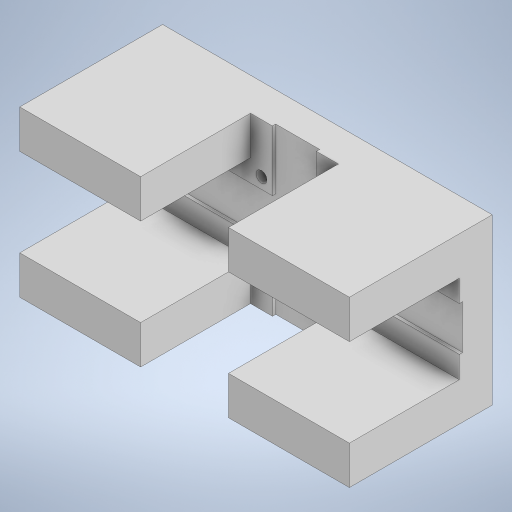
# Autodesk Inventor part: Bauteil1
Saved by Autodesk Inventor 2024 (Build 280153000, 153)
## iProperties
Created: 2023-11-13
Part Number: Bauteil1
Material: Generisch
Document SubType Name: Modeling
Designer: Luca
Density: 1 g/cm^3
Appearance: Vorgabe
Author: Luca
Autodesk Inventor part; units mm, degrees
ref_plane "YZ Plane" through (0, 0, 0) normal (1, 0, 0) x (0, 1, 0)
ref_plane "XZ Plane" through (0, 0, 0) normal (0, 1, 0) x (-1, 0, 0)
ref_plane "XY Plane" through (0, 0, 0) normal (0, 0, 1) x (1, 0, 0)
sketch "Skizze2" plane through (0, 0, 0) normal (0, 0, 1) x (1, 0, 0)
  line L0 (-30.3771, 139.6504) -> (269.6229, 139.6504)
  line L1 (269.6229, 139.6504) -> (269.6229, -10.3496)
  line L2 (269.6229, -10.3496) -> (-30.3771, -10.3496)
  line L3 (-30.3771, -10.3496) -> (-30.3771, 139.6504)
  point P0 (0, 0)
  dimension "d4" = 300
  dimension "d5" = 150
  constraints: 8 end point, 2 parallel, 1 horizontal, 1 perpendicular
  measures "d4" distance of L1.end L2.end
  measures "d5" distance between parallel lines of L2 L0
extrude "Extrusion2" add sketch "Skizze2" along normal blind 30
sketch "Skizze3" plane through (0, 0, 30) normal (0, 0, 1) x (1, 0, 0)
  line L0 (-30.3771, 139.6504) -> (-30.3771, -10.3496) projected
  line L1 (269.6229, -10.3496) -> (269.6229, 139.6504) projected
  line L2 (-30.3771, 84.6504) -> (269.6229, 84.6504)
  line L3 (269.6229, 84.6504) -> (269.6229, 44.6504)
  line L4 (269.6229, 44.6504) -> (-30.3771, 44.6504)
  line L5 (-30.3771, 44.6504) -> (-30.3771, 84.6504)
  line L6 (269.6229, 139.6504) -> (-30.3771, 139.6504) projected
  point P0 (0, 0)
  dimension "d8" = 40
  dimension "d9" = 55
  constraints: 8 end point, 2 parallel, 2 point on line, 1 horizontal, 1 perpendicular
  measures "d8" distance of L2.end L3.end
  measures "d9" distance between parallel lines of L2 L6
extrude "Extrusion3" cut sketch "Skizze3" against normal blind 3 contours L2 L1 L4 L0
sketch "Skizze5" plane through (0, 0, 30) normal (0, 0, 1) x (1, 0, 0)
  line L0 (-30.3771, -10.3496) -> (269.6229, -10.3496) projected
  line L1 (269.6229, 139.6504) -> (-30.3771, 139.6504) projected
  line L2 (99.6229, -10.3496) -> (139.6229, -10.3496)
  line L3 (139.6229, -10.3496) -> (139.6229, 139.6504)
  line L4 (139.6229, 139.6504) -> (99.6229, 139.6504)
  line L5 (99.6229, 139.6504) -> (99.6229, -10.3496)
  line L6 (-30.3771, 139.6504) -> (-30.3771, 84.6504) projected
  point P0 (0, 0)
  dimension "d15" = 40
  dimension "d16" = 130
  constraints: 8 end point, 2 parallel, 2 point on line, 1 horizontal, 1 perpendicular
  measures "d15" distance of L4.end L3.end
  measures "d16" distance between parallel lines of L5 L6
extrude "Extrusion4" cut sketch "Skizze5" against normal blind 3
sketch "Skizze6" plane through (0, 0, 30) normal (0, 0, 1) x (1, 0, 0)
  line L0 (-30.3771, 139.6504) -> (-30.3771, -10.3496) projected
  line L1 (-30.3771, 139.6504) -> (79.6229, 139.6504)
  line L2 (79.6229, 139.6504) -> (79.6229, 104.6504)
  line L3 (79.6229, 104.6504) -> (-30.3771, 104.6504)
  line L4 (-30.3771, 104.6504) -> (-30.3771, 139.6504)
  line L5 (269.6229, 139.6504) -> (139.6229, 139.6504) projected
  line L6 (269.6229, 139.6504) -> (159.6229, 139.6504)
  line L7 (159.6229, 139.6504) -> (159.6229, 104.6504)
  line L8 (159.6229, 104.6504) -> (269.6229, 104.6504)
  line L9 (269.6229, 104.6504) -> (269.6229, 139.6504)
  line L10 (269.6229, -10.3496) -> (269.6229, 44.6504) projected
  line L11 (269.6229, -10.3496) -> (159.6229, -10.3496)
  line L12 (159.6229, -10.3496) -> (159.6229, 24.6504)
  line L13 (159.6229, 24.6504) -> (269.6229, 24.6504)
  line L14 (269.6229, 24.6504) -> (269.6229, -10.3496)
  line L15 (-30.3771, -10.3496) -> (79.6229, -10.3496)
  line L16 (79.6229, -10.3496) -> (79.6229, 24.6504)
  line L17 (79.6229, 24.6504) -> (-30.3771, 24.6504)
  line L18 (-30.3771, 24.6504) -> (-30.3771, -10.3496)
  point P0 (0, 0)
  dimension "d19" = 110
  dimension "d20" = 35
  dimension "d21" = 110
  dimension "d22" = 35
  dimension "d23" = 110
  dimension "d24" = 35
  dimension "d25" = 110
  dimension "d26" = 35
  constraints: 32 end point, 8 parallel, 4 horizontal, 4 perpendicular
  measures "d19" distance of L2.end L3.end
  measures "d20" distance of L1.end L2.end
  measures "d21" distance of L8.end L7.end
  measures "d22" distance of L7.end L6.end
  measures "d23" distance of L12.end L13.end
  measures "d24" distance of L11.end L12.end
  measures "d25" distance of L17.end L16.end
  measures "d26" distance of L16.end L15.end
extrude "Extrusion5" add sketch "Skizze6" along normal blind 100
sketch "Skizze7" plane through (0, 0, 0) normal (0, 0, -1) x (-1, 0, 0)
  line L0 (20.3771, -0.3496) -> (-259.6229, -0.3496)
  line L1 (-259.6229, -0.3496) -> (-259.6229, 129.6504)
  line L2 (-259.6229, 129.6504) -> (20.3771, 129.6504)
  line L3 (20.3771, 129.6504) -> (20.3771, -0.3496)
  line L4 (30.3771, -10.3496) -> (-269.6229, -10.3496) projected
  line L5 (30.3771, 139.6504) -> (30.3771, -10.3496) projected
  line L6 (-234.6229, -10.3496) -> (-244.6229, -10.3496)
  line L7 (-244.6229, -10.3496) -> (-244.6229, -0.3496)
  line L8 (-244.6229, -0.3496) -> (-234.6229, -0.3496)
  line L9 (-234.6229, -0.3496) -> (-234.6229, -10.3496)
  line L10 (-269.6229, -10.3496) -> (-269.6229, 139.6504) projected
  point P0 (0, 0)
  point P1 (-239.6229, -10.3496)
  point P2 (-244.6229, -5.3496)
  dimension "d29" = 280
  dimension "d30" = 130
  dimension "d31" = 10
  dimension "d32" = 10
  dimension "d33" = 10
  dimension "d34" = 10
  dimension "d36" = 0
  dimension "d37" = 25
  constraints: 16 end point, 4 parallel, 2 horizontal, 2 midpoint, 2 perpendicular
  measures "d29" distance of L1.end L2.end
  measures "d30" distance of L0.end L1.end
  measures "d31" distance between parallel lines of L0 L4
  measures "d32" distance between parallel lines of L5 L3
  measures "d33" distance of L7.end L8.end
  measures "d34" distance of L6.end L7.end
  measures "d36" distance from line of L4 point (-239.623, -10.35)
  measures "d37" distance from line of L10 point (-244.623, -5.35)
extrude "Extrusion6" cut sketch "Skizze7" against normal blind 20
sketch "Skizze8" plane through (0, 0, 30) normal (0, 0, 1) x (1, 0, 0)
  circle A0 centre (89.6229, 94.6504) radius 5
  line L0 (-30.3771, 84.6504) -> (99.6229, 84.6504) projected
  line L1 (99.6229, 84.6504) -> (99.6229, 139.6504) projected
  circle A1 centre (89.6229, 34.6504) radius 5
  line L2 (99.6229, 44.6504) -> (-30.3771, 44.6504) projected
  line L3 (99.6229, -10.3496) -> (99.6229, 44.6504) projected
  circle A2 centre (149.6229, 34.6504) radius 5
  line L4 (139.6229, 44.6504) -> (139.6229, -10.3496) projected
  circle A3 centre (149.6229, 94.6504) radius 5
  line L5 (139.6229, 139.6504) -> (139.6229, 84.6504) projected
  point P0 (0, 0)
  dimension "d40" = 10
  dimension "d41" = 10
  dimension "d42" = 10
  dimension "d43" = 10
  dimension "d44" = 10
  dimension "d45" = 10
  dimension "d46" = 10
  dimension "d47" = 10
  dimension "d48" = 10
  dimension "d49" = 10
  constraints: 4 centre point
  measures "d40" diameter of A0
  measures "d41" distance from line of A0.centre L0
  measures "d42" distance from line of A0.centre L1
  measures "d43" diameter of A1
  measures "d44" distance from line of L2 A1.centre
  measures "d45" distance from line of L3 A1.centre
  measures "d46" diameter of A2
  measures "d47" distance from line of L4 A2.centre
  measures "d48" diameter of A3
  measures "d49" distance from line of L5 A3.centre
extrude "Extrusion7" cut sketch "Skizze8" against normal through all
